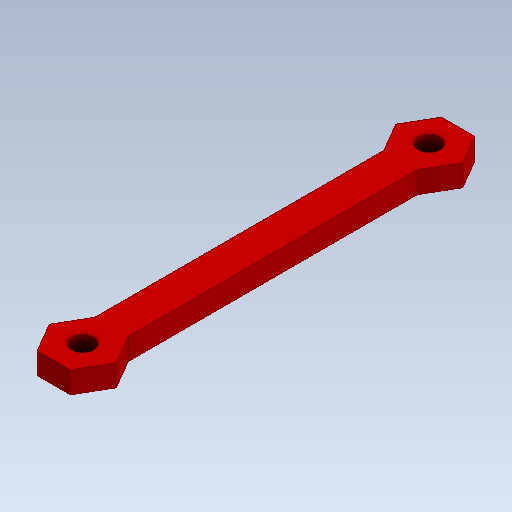
# Autodesk Inventor part: HexServoCover
Saved by Autodesk Inventor 2020 (Build 240168000, 168)
## iProperties
Created: 2023-12-27
Part Number: HexServoCover
Material: PETG
Document SubType Name: Modeling
Designer: smz3rm
Density: 1 g/cm^3
Appearance: Generic
Mass: 0.841524 g
Surface Area: 9.98014 cm^2
Volume: 0.841524 cm^3
Author: smz3rm
Autodesk Inventor part; units mm, degrees
ref_plane "YZ Plane" through (0, 0, 0) normal (1, 0, 0) x (0, 1, 0)
ref_plane "XZ Plane" through (0, 0, 0) normal (0, 1, 0) x (-1, 0, 0)
ref_plane "XY Plane" through (0, 0, 0) normal (0, 0, 1) x (1, 0, 0)
sketch "Sketch1" plane through (0, 0, 0) normal (0, 1, 0) x (-1, 0, 0)
  line L0 (-2.3094, 20) -> (2.3094, 20)
  line L1 (2.3094, 20) -> (2.3094, -20)
  line L2 (2.3094, -20) -> (-2.3094, -20)
  line L3 (-2.3094, -20) -> (-2.3094, 20)
  line L4 (-2.3094, 20) -> (2.3094, -20) construction
  line L5 (2.3094, 20) -> (-2.3094, -20) construction
  line L6 (-2.3094, -20) -> (2.3094, -20)
  line L7 (2.3094, -20) -> (4.6188, -24)
  line L8 (4.6188, -24) -> (2.3094, -28)
  line L9 (2.3094, -28) -> (-2.3094, -28)
  line L10 (-2.3094, -28) -> (-4.6188, -24)
  line L11 (-4.6188, -24) -> (-2.3094, -20)
  line L12 (0, -39.2) -> (0, 39.2) projected
  line L13 (6.4663, 0) -> (-6.4663, 0) projected
  line L14 (2.3094, 20) -> (-2.3094, 20)
  line L15 (-2.3094, 20) -> (2.3094, 20)
  line L16 (2.3094, 20) -> (4.6188, 24)
  line L17 (4.6188, 24) -> (2.3094, 28)
  line L18 (2.3094, 28) -> (-2.3094, 28)
  line L19 (-2.3094, 28) -> (-4.6188, 24)
  line L20 (-4.6188, 24) -> (-2.3094, 20)
  circle A0 centre (0, -24) radius 1.55
  circle A1 centre (0, 24) radius 1.55
  point P0 (0, 0)
  point P1 (-2.3094, 20)
  point P2 (-2.3094, -20)
  dimension "d1" = 40
  dimension "d2" = 8
  dimension "d3" = 3.1
  dimension "d4" = 3.1
  constraints: 40 end point, 7 symmetric about line, 3 point on line, 2 centre point, 2 coincident, 2 midpoint, 2 parallel, 1 horizontal, 1 perpendicular, 13 other
  measures "d1" distance of L1.end L0.end
  measures "d2" distance between parallel lines of L2 L9
  measures "d3" diameter of A0
  measures "d4" diameter of A1
extrude "Extrusion1" add sketch "Sketch1" along normal blind 3 contours L20 L19 L18 L12 A1 L0 | L0 L12 L13 L3 | L12 A1 L18 L17 L16 L0 | L0 L1 L13 L12 | L13 L12 L2 L3 | L13 L1 L2 L12 | L2 L12 A0 L9 L10 L11 | L2 L7 L8 L9 L12 A0
equation "\"d2\" = M3ScrewInsertBrim"
equation "\"d3\" = M3ScrewDia"
equation "\"d4\" = M3ScrewDia"
equation "\"M3ScrewInsertBrim\" = 8"
equation "\"M3ScrewDia\" = 3.1"
body "Solid1"
